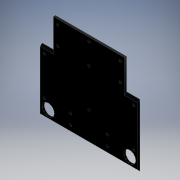
# Autodesk Inventor part: Podstawa
Saved by Autodesk Inventor 2017 (Build 210142000, 142)
## iProperties
Created: 2016-11-09
Part Number: Podstawa
Material: Generic
Document SubType Name: Modeling
Designer: Shichi
Density: 1 g/cm^3
Appearance: Gunmetal - Polished
Author: Shichi
Autodesk Inventor part; units mm, degrees
ref_plane "YZ Plane" through (0, 0, 0) normal (1, 0, 0) x (0, 1, 0)
ref_plane "XZ Plane" through (0, 0, 0) normal (0, 1, 0) x (-1, 0, 0)
ref_plane "XY Plane" through (0, 0, 0) normal (0, 0, 1) x (1, 0, 0)
sketch "Sketch1" plane through (0, 0, 0) normal (0, 1, 0) x (-1, 0, 0)
  line L0 (35, 45.5) -> (35, 15.5)
  line L1 (9, 15.5) -> (35, 15.5) construction
  line L2 (0, 15.5) -> (9, 15.5) construction
  line L3 (35, 15.5) -> (48, 15.5)
  line L4 (0, -45.5) -> (0, 45.5)
  line L5 (0, -45.5) -> (48, -45.5)
  line L6 (0, 45.5) -> (35, 45.5)
  line L7 (48, -45.5) -> (48, 15.5)
  line L8 (30.7, 40.55) -> (35, 40.55) construction
  line L9 (30.7, 40.55) -> (30.7, 22.45) construction
  circle A0 centre (30.7, 22.45) radius 1.25
  circle A1 centre (30.7, 40.55) radius 1.25
  line L10 (30.7, 22.45) -> (30.7, 15.5) construction
  line L11 (44, 15.5) -> (44, 9.5) construction
  line L12 (44, 9.5) -> (48, 9.5) construction
  circle A2 centre (44, 9.5) radius 1.25
  circle A3 centre (44, -28.5) radius 1.25
  circle A4 centre (18, -28.5) radius 1.25
  circle A5 centre (18, -38.5) radius 1.25
  arc A6 (0, -17.75) -> (0, -15.25) centre (0, -16.5) ccw
  arc A7 (0, 40.55) -> (0, 43.05) centre (0, 41.8) ccw
  arc A8 (0, 19.95) -> (0, 22.45) centre (0, 21.2) ccw
  line L13 (0, 41.8) -> (30.7, 41.8) construction
  line L14 (0, 21.2) -> (30.7, 21.2) construction
  circle A9 centre (40, -36.5) radius 6
  point P0 (0, 0)
  point P1 (-50, 0)
  point P2 (0, 0)
  dimension "d16" = 2.5
  dimension "d17" = 2.5
  dimension "d6" = 30
  dimension "d9" = 26
  dimension "d10" = 9
  dimension "d11" = 48
  dimension "d12" = 91
  dimension "d14" = 4.3
  dimension "d15" = 18.1
  dimension "d20" = 6.95
  dimension "d25" = 6
  dimension "d26" = 4
  dimension "d27" = 2.5
  dimension "d30" = 2.5
  dimension "d32" = 2.5
  dimension "d33" = 18
  dimension "d34" = 2.5
  dimension "d35" = 10
  dimension "d36" = 2.5
  dimension "d37" = 2.5
  dimension "d38" = 1.25
  dimension "d42" = 12
  dimension "d43" = 8
  dimension "d45" = 26
  dimension "d46" = 46
  dimension "d47" = 38
  constraints: 28 end point, 10 vertical alignment, 8 centre point, 7 horizontal alignment, 6 point on circle, 5 horizontal, 5 point on line, 4 coincident, 2 perpendicular, 2 vertical, 1 parallel, 17 other
  measures "d6" distance of L0.start L0.end
  measures "d9" distance of L1.start L0.end
  measures "d10" distance of L2.start L1.start
  measures "d11" distance of L5.start L5.end
  measures "d12" distance of L5.start L6.start
  measures "d14" distance of L8.start L8.end
  measures "d15" distance of L8.start L9.end
  measures "d20" distance of L10.start L10.end
  measures "d25" distance of L11.start L11.end
  measures "d26" distance of L11.end L12.end
  measures "d27" diameter of A2
  measures "d30" diameter of A3
  measures "d32" diameter of A4
  measures "d34" diameter of A5
  measures "d35" distance of A5.centre A4.centre
  measures "d36" diameter of A6
  measures "d37" diameter of A8
  measures "d38" radius of A7
  measures "d42" diameter of A9
  measures "d43" distance from line of A9.centre L7
  measures "d45" vertical distance of A2.centre A6.centre
  measures "d46" vertical distance of A2.centre A9.centre
  measures "d47" distance of L11.end A3.centre
extrude "Extrusion1" add sketch "Sketch1" along normal blind 2 contours L0 L3 L7 L5 L4 A6 A8 A7 L6 | A7 L4 | A8 L4 | L4 A6 | A0 | A1 | A2 | A3 | A4 | A5 | A9
extrude "Extrusion2" cut sketch "Sketch1" along normal through all contours A7 L4 | A8 L4 | L4 A6 | A0 | A1 | A2 | A3 | A4 | A5 | A9
mirror "Mirror1" about plane through (0, 0, 0) normal (1, 0, 0) of "Extrusion1", "Extrusion2"
sketch "Sketch3" plane through (0, 0, 0) normal (1, 0, 0) x (0, 1, 0)
  line L0 (0, 15.5) -> (0, -45.5) projected
  line L1 (0, -45.5) -> (2, -45.5) projected
  line L2 (0, -45.5) -> (2, -45.5)
  line L3 (2, -45.5) -> (0, -43.5)
  line L4 (0, -43.5) -> (0, -45.5)
  line L5 (2, -45.5) -> (2, 15.5) projected
  point P0 (0, 0)
  dimension "d24" = 45
  constraints: 6 end point, 2 collinear, 1 point on line
  measures "d24" angle of L5 L3
extrude "Extrusion3" cut sketch "Sketch3" along normal through all both and the other way through all
chamfer "Chamfer1" distance 2 angle 45 2 edges at (-41.5, 0, 15.5) (41.5, 0, 15.5)
body "Solid1"
